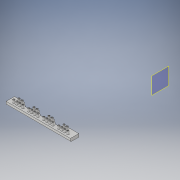
# Autodesk Inventor part: Part2
Saved by Autodesk Inventor 2019 (Build 230136000, 136)
## iProperties
Created: 2020-09-08
Part Number: Part2
Material: Generic
Document SubType Name: Modeling
Designer: Sergio
Density: 1 g/cm^3
Appearance: Default
Author: Sergio
Autodesk Inventor part; units mm, degrees
ref_plane "YZ Plane" through (0, 0, 0) normal (1, 0, 0) x (0, 1, 0)
ref_plane "XZ Plane" through (0, 0, 0) normal (0, 1, 0) x (-1, 0, 0)
ref_plane "XY Plane" through (0, 0, 0) normal (0, 0, 1) x (1, 0, 0)
sketch "Sketch1" plane through (0, 0, 0) normal (0, 1, 0) x (-1, 0, 0)
  circle A0 centre (41.3055, -60.0191) radius 0.95
  circle A1 centre (39.0419, -55.5191) radius 0.95
  circle A2 centre (35.0419, -55.5191) radius 0.95
  circle A3 centre (37.3055, -60.0191) radius 0.95
  circle A4 centre (33.3055, -60.0191) radius 0.95
  circle A5 centre (29.3055, -60.0191) radius 0.95
  circle A6 centre (13.8055, -60.0191) radius 0.95
  circle A7 centre (15.5419, -55.5191) radius 0.95
  circle A8 centre (17.8055, -60.0191) radius 0.95
  circle A9 centre (19.5419, -55.5191) radius 0.95
  circle A10 centre (9.8055, -60.0191) radius 0.95
  circle A11 centre (0.0419, -55.5191) radius 0.95
  circle A12 centre (2.3055, -60.0191) radius 0.95
  circle A13 centre (-5.6945, -60.0191) radius 0.95
  circle A14 centre (-1.6945, -60.0191) radius 0.95
  circle A15 centre (-9.6945, -60.0191) radius 0.95
  circle A16 centre (-3.9581, -55.5191) radius 0.95
  circle A17 centre (-23.4581, -55.5191) radius 0.95
  circle A18 centre (-29.1945, -60.0191) radius 0.95
  circle A19 centre (-19.4581, -55.5191) radius 0.95
  circle A20 centre (-21.1945, -60.0191) radius 0.95
  circle A21 centre (-17.1945, -60.0191) radius 0.95
  circle A22 centre (-25.1945, -60.0191) radius 0.95
  circle A23 centre (21.8055, -60.0191) radius 0.95
  line L0 (39.0419, -52.5191) -> (41.3055, -48.7591)
  line L1 (41.3055, -48.7591) -> (41.3055, -46.2591)
  line L2 (41.3055, -46.2591) -> (47.8055, -46.2591)
  line L3 (19.5419, -52.5191) -> (15.5419, -52.5191)
  line L4 (9.8055, -57.0191) -> (15.5419, -52.5191)
  line L5 (0.0419, -52.5191) -> (-3.9581, -52.5191)
  line L6 (-9.6945, -57.0191) -> (-3.9581, -52.5191)
  line L7 (-35.6945, -52.5191) -> (-19.4581, -52.5191)
  line L8 (-29.1945, -63.4191) -> (41.3055, -63.4191) construction
  line L9 (-35.6945, -63.4191) -> (47.8055, -63.4191)
  line L10 (47.8055, -63.4191) -> (47.8055, -46.2591)
  line L11 (29.3055, -57.0191) -> (24.3055, -57.0191)
  line L12 (24.3055, -57.0191) -> (19.5419, -52.5191)
  line L13 (9.8055, -57.0191) -> (4.8055, -57.0191)
  line L14 (4.8055, -57.0191) -> (0.0419, -52.5191)
  line L15 (-9.6945, -57.0191) -> (-14.6945, -57.0191)
  line L16 (-14.6945, -57.0191) -> (-19.4581, -52.5191)
  line L17 (47.8055, -52.5191) -> (35.0419, -52.5191)
  line L18 (35.0419, -52.5191) -> (29.3055, -57.0191)
  line L19 (-26.9309, -52.5191) -> (-29.1945, -48.7591)
  line L20 (-29.1945, -48.7591) -> (-29.1945, -46.2591)
  line L21 (-29.1945, -46.2591) -> (-35.6945, -46.2591)
  line L22 (-35.6945, -63.4191) -> (-35.6945, -46.2591)
  point P0 (0, 0)
  point P1 (0, 0)
  point P2 (0, 0)
  dimension "d2" = 1.9
  dimension "d3" = 1.9
  dimension "d4" = 1.9
  dimension "d5" = 1.9
  dimension "d7" = 1.9
  dimension "d9" = 1.9
  dimension "d10" = 1.9
  dimension "d11" = 1.9
  dimension "d12" = 1.9
  dimension "d13" = 1.9
  dimension "d14" = 1.9
  dimension "d15" = 1.9
  dimension "d16" = 1.9
  dimension "d18" = 1.9
  dimension "d19" = 1.9
  dimension "d20" = 1.9
  dimension "d21" = 1.9
  dimension "d22" = 1.9
  dimension "d23" = 1.9
  dimension "d54" = 1.9
  dimension "d55" = 1.9
  dimension "d56" = 1.9
  dimension "d57" = 1.9
  dimension "d58" = 1.9
  constraints: 46 end point, 24 centre point, 6 horizontal, 4 point on line, 3 vertical, 1 perpendicular
  measures "d2" diameter of A0
  measures "d3" diameter of A3
  measures "d4" diameter of A5
  measures "d5" diameter of A4
  measures "d7" diameter of A9
  measures "d9" diameter of A8
  measures "d10" diameter of A7
  measures "d11" diameter of A10
  measures "d12" diameter of A6
  measures "d13" diameter of A11
  measures "d14" diameter of A12
  measures "d15" diameter of A14
  measures "d16" diameter of A13
  measures "d18" diameter of A19
  measures "d19" diameter of A21
  measures "d20" diameter of A20
  measures "d21" diameter of A17
  measures "d22" diameter of A18
  measures "d23" diameter of A22
  measures "d54" diameter of A1
  measures "d55" diameter of A2
  measures "d56" diameter of A23
  measures "d57" diameter of A15
  measures "d58" diameter of A16
extrude "Extrusion1" add sketch "Sketch1" against normal blind 4 contours L17 L10 L9 L22 L7 L16 L15 L6 L5 L14 L13 L4 L3 L12 L11 L18
sketch "Sketch2" plane through (0, 0, 0) normal (0, 1, 0) x (1, 0, 0)
  circle A0 centre (29.1945, 60.0191) radius 0.95 projected
  line L0 (29.1945, 60.0191) -> (28.2445, 60.0191)
  circle A1 centre (25.1945, 60.0191) radius 0.95 projected
  circle A2 centre (23.4581, 55.5191) radius 0.95 projected
  circle A3 centre (21.1945, 60.0191) radius 0.95 projected
  circle A4 centre (19.4581, 55.5191) radius 0.95 projected
  circle A5 centre (17.1945, 60.0191) radius 0.95 projected
  circle A6 centre (9.6945, 60.0191) radius 0.95 projected
  circle A7 centre (5.6945, 60.0191) radius 0.95 projected
  circle A8 centre (3.9581, 55.5191) radius 0.95 projected
  circle A9 centre (-0.0419, 55.5191) radius 0.95 projected
  circle A10 centre (1.6945, 60.0191) radius 0.95 projected
  circle A11 centre (-2.3055, 60.0191) radius 0.95 projected
  circle A12 centre (-21.8055, 60.0191) radius 0.95 projected
  circle A13 centre (-17.8055, 60.0191) radius 0.95 projected
  circle A14 centre (-13.8055, 60.0191) radius 0.95 projected
  circle A15 centre (-9.8055, 60.0191) radius 0.95 projected
  circle A16 centre (-15.5419, 55.5191) radius 0.95 projected
  circle A17 centre (-19.5419, 55.5191) radius 0.95 projected
  circle A18 centre (-37.3055, 60.0191) radius 0.95 projected
  circle A19 centre (-33.3055, 60.0191) radius 0.95 projected
  circle A20 centre (-29.3055, 60.0191) radius 0.95 projected
  circle A21 centre (-35.0419, 55.5191) radius 0.95 projected
  circle A22 centre (-39.0419, 55.5191) radius 0.95 projected
  circle A23 centre (-41.3055, 60.0191) radius 0.95 projected
  point P0 (0, 0)
  constraints: 23 coincident, 2 end point, 1 horizontal alignment, 1 other
ref_plane "Work Plane1" through (29.1945, 0, -60.0191) normal (-1, 0, 0) x (0, -1, 0)
sketch "Sketch3" plane through (29.1945, 0, -60.0191) normal (-1, 0, 0) x (0, -1, 0)
  line L0 (0, 0) -> (4, 0) construction
  line L1 (0, 0.95) -> (-4, 0.95)
  line L2 (-4, 0.95) -> (-4, 1.25)
  line L3 (-4, 1.25) -> (0, 1.25)
  line L4 (0, 1.25) -> (0, 0.95)
  line L5 (-4, 0.95) -> (-4, 0.65)
  line L6 (-4, 0.95) -> (-3.8, 0.95)
  line L7 (-3.8, 0.95) -> (-4, 0.65)
  line L8 (-3.8, 0.95) -> (-2.6, 0.95) construction
  line L9 (-2.6, 0.95) -> (-2.6, 0.65)
  line L10 (-2.6, 0.95) -> (-2.4, 0.95)
  line L11 (-2.4, 0.95) -> (-2.6, 0.65)
  line L12 (-2.4, 0.95) -> (-1.2, 0.95) construction
  line L13 (-1.2, 0.95) -> (-1.2, 0.65)
  line L14 (-1.2, 0.95) -> (-1, 0.95)
  line L15 (-1, 0.95) -> (-1.2, 0.65)
  point P0 (0, 60.0191)
  point P1 (0, -0.95)
  point P2 (4, 0.95)
  dimension "d81" = 4
  dimension "d92" = 0.3
  dimension "d93" = 0.2
  dimension "d94" = 1.2
  dimension "d95" = 0.3
  dimension "d96" = 0.2
  dimension "d97" = 1.2
  dimension "d98" = 0.3
  dimension "d99" = 0.2
  constraints: 32 end point, 5 point on line, 3 vertical, 2 parallel, 1 horizontal, 1 perpendicular
  measures "d81" distance of L2.end L3.end
  measures "d92" distance of L1.end L5.end
  measures "d93" distance of L1.end L6.end
  measures "d94" distance of L6.end L8.end
  measures "d95" distance of L8.end L9.end
  measures "d96" distance of L8.end L10.end
  measures "d97" distance of L10.end L12.end
  measures "d98" distance of L12.end L13.end
  measures "d99" distance of L12.end L14.end
fillet "Fillet4" radius 1 1 edges at (-6.0555, -4, -63.4191)
revolve "Revolution3" add sketch "Sketch3" angle 360 about axis through (29.1945, 0, -60.0191) along (0, -1, 0)
fillet "Fillet5" radius 0.5 1 edges at (29.1945, 4, -61.2691)
pattern_sketch "Sketch Driven Pattern4" of "Fillet5", "Revolution3" from (29.1945, 0, -60.0191) copies at (25.1945, 0, -60.0191) at (23.4581, 0, -55.5191) at (21.1945, 0, -60.0191) at (19.4581, 0, -55.5191) at (17.1945, 0, -60.0191) at (9.6945, 0, -60.0191) at (5.6945, 0, -60.0191) at (3.9581, 0, -55.5191) at (-0.0419, 0, -55.5191) at (1.6945, 0, -60.0191) at (-2.3055, 0, -60.0191) at (-21.8055, 0, -60.0191) at (-17.8055, 0, -60.0191) at (-13.8055, 0, -60.0191) at (-9.8055, 0, -60.0191) at (-15.5419, 0, -55.5191) at (-19.5419, 0, -55.5191) at (-37.3055, 0, -60.0191) at (-33.3055, 0, -60.0191) at (-29.3055, 0, -60.0191) at (-35.0419, 0, -55.5191) at (-39.0419, 0, -55.5191) at (-41.3055, 0, -60.0191)
mirror "Mirror3" about plane through (0, 0, 0) normal (0, 0, 1) remove original yes
body "Solid1"
